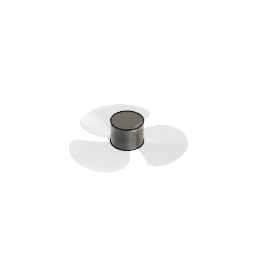
day25-surface-propeller (Autodesk Fusion 360 design; units mm, degrees)
part number: 2026-06-16-11-28-33-197
part number: 2026-06-16-11-30-40-811
Autodesk Fusion 360 part; units mm, degrees
sketch "Sketch1" plane through (0, 0, 0) normal (0, 0, 1) x (1, 0, 0) in component "Propeller"
  circle A0 centre (0, 0) radius 20
  dimension "d1" = 40
  constraint coincident A0.centre origin
  measures "d1" diameter of A0
extrude "Extrude1" add sketch "Sketch1" along normal blind 30 in component "Propeller"
ref_plane "WorkPlane1" through (0, -12, 0) normal (0, 1, 0) x (0, 0, 1) in component "Propeller"
ref_plane "WorkPlane2" through (0, -112, 0) normal (0, 1, 0) x (0, 0, 1) in component "Propeller"
sketch "Sketch2" plane through (0, -112, 0) normal (0, 1, 0) x (1, 0, 0) in component "Propeller"
component "Propeller" placed x (1, 0, 0) y (0, 1, 0) z (0, 0, 1) at (0, 0, 0)
